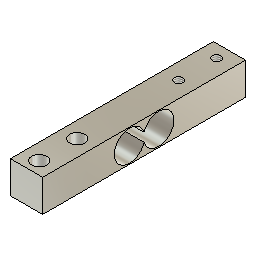
vibroDoser (Autodesk Fusion 360 archive; units mm, degrees)
design "LoadCell"
Autodesk Fusion 360 part; units mm, degrees
(part 1 of 2)
sketch "Skizze2" plane through (0, 0, 0) normal (0, 1, 0) x (1, 0, 0)
  line L0 (-6.35, -6.35) -> (6.35, -6.35)
  line L1 (6.35, -6.35) -> (6.35, 6.35)
  line L2 (6.35, 6.35) -> (-6.35, 6.35)
  line L3 (-6.35, 6.35) -> (-6.35, -6.35)
  line L4 (-6.35, -6.35) -> (6.35, 6.35) construction
  line L5 (6.35, -6.35) -> (-6.35, 6.35) construction
  dimension "d1" = 12.7
  dimension "d2" = 12.7
  constraint horizontal L0
  constraint perpendicular L0 L1
  constraint parallel L0 L2
  constraint parallel L1 L3
  constraint coincident L4 origin
  constraint coincident L5 origin
  measures "d1" distance of L1.end L2.end
  measures "d2" distance of L0.end L1.end
extrude "Extrusion1" add sketch "Skizze2" along normal blind 80
sketch "Skizze3" plane through (6.35, 0, 0) normal (1, 0, 0) x (0, 1, 0)
  line L0 (0, 6.35) -> (0, -6.35)
  line L1 (0, -6.35) -> (80, -6.35)
  line L2 (80, -6.35) -> (80, 6.35)
  line L3 (80, 6.35) -> (0, 6.35)
  line L4 (0, 0) -> (85.7645, 0) construction
  circle A0 centre (34.25, 0) radius 6
  circle A1 centre (45.75, 0) radius 6
  line L5 (40, -6.35) -> (40, 14.7485) construction
  dimension "d5" = 11.5
  dimension "d6" = 12
  dimension "d7" = 12
  dimension "d8" = 5.75
  constraint coincident L4.start origin
  constraint perpendicular L0 L4
  constraint coincident L4 A0.centre
  constraint coincident L4 A1.centre
  constraint midpoint L1 L5.start
  constraint perpendicular L3 L5
  measures "d5" distance of A0.centre A1.centre
  measures "d6" diameter of A1
  measures "d7" diameter of A0
  measures "d8" distance of A0.centre L5
extrude "Extrusion2" cut sketch "Skizze3" against normal blind 27 contours A0 A1 | A0 A1 | A0 A1
sketch "Skizze4" plane through (0, 0, 6.35) normal (0, 0, 1) x (-1, 0, 0)
  line L0 (6.35, 0) -> (-6.35, 0)
  line L1 (-6.35, 0) -> (-6.35, -80)
  line L2 (-6.35, -80) -> (6.35, -80)
  line L3 (6.35, -80) -> (6.35, 0)
  line L4 (0, 5.2844) -> (0, -87.2424)
  point P0 (0, -5)
  point P1 (0, -20)
  point P2 (0, -60)
  point P3 (0, -75)
  dimension "d11" = 5
  dimension "d12" = 15
  dimension "d13" = 15
  dimension "d14" = 5
  constraint perpendicular L2 L4
  constraint coincident origin L4
  constraint coincident L4 P0
  constraint coincident L4 P1
  constraint coincident L4 P2
  constraint coincident L4 P3
  measures "d11" distance of L0 P0
  measures "d12" distance of P0 P1
  measures "d13" distance of P2 P3
  measures "d14" distance of L2 P3
hole "Bohrung1" at (0, 5, 6.35) at (0, 20, 6.35) direction (0, 0, -1) diameter 6 depth 30 tip angle 118
hole "Bohrung2" at (0, 60, 6.35) at (0, 75, 6.35) direction (0, 0, -1) diameter 3.332 depth 30 tip angle 118
thread "Gewinde2" "ISO Metric profile 4.0 M4x0.7 6H"
equation "d8 = ( 11.5 / 2 ) * 1 mm"

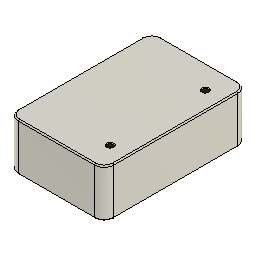
design "Schaltschrank"
Autodesk Fusion 360 part; units mm, degrees
sketch "Skizze1" plane through (0, 0, 0) normal (0, 0, 1) x (1, 0, 0)
  line L0 (-200, 300) -> (200, 300)
  line L1 (200, 300) -> (200, -300)
  line L2 (200, -300) -> (-200, -300)
  line L3 (-200, -300) -> (-200, 300)
  line L4 (-200, 300) -> (200, -300) construction
  line L5 (200, 300) -> (-200, -300) construction
  dimension "d1" = 600
  dimension "d2" = 400
  constraint horizontal L0
  constraint perpendicular L0 L1
  constraint parallel L0 L2
  constraint parallel L1 L3
  constraint coincident L4 origin
  constraint coincident L5 origin
  measures "d1" distance of L0.end L1.end
  measures "d2" distance of L0.start L0.end
extrude "Extrusion1" add sketch "Skizze1" along normal blind 200
fillet "Abrundung1" radius 40 4 edges at (200, -300, 100) (-200, -300, 100) (200, 300, 100) (-200, 300, 100)
fillet "Abrundung2" radius 5 2 faces at (-66.6667, -86.6667, 200) (-66.6667, -86.6667, 0)
sketch "Skizze2" plane through (0, 0, 200) normal (0, 0, 1) x (-1, 0, 0)
  arc A0 (160, -295) -> (195, -260) centre (160, -260) ccw
  line L0 (195, -260) -> (195, 260)
  arc A1 (195, 260) -> (160, 295) centre (160, 260) ccw
  line L1 (160, 295) -> (-160, 295)
  arc A2 (-160, 295) -> (-195, 260) centre (-160, 260) ccw
  line L2 (-195, 260) -> (-195, -260)
  arc A3 (-195, -260) -> (-160, -295) centre (-160, -260) ccw
  line L3 (-160, -295) -> (160, -295)
  line L4 (-125, -200) -> (125, -200)
  line L5 (125, -200) -> (125, 200)
  line L6 (125, 200) -> (-125, 200)
  line L7 (-125, 200) -> (-125, -200)
  line L8 (-125, -200) -> (125, 200) construction
  line L9 (125, -200) -> (-125, 200) construction
  dimension "d9" = 250
  dimension "d10" = 400
  constraint horizontal L4
  constraint perpendicular L4 L5
  constraint parallel L4 L6
  constraint parallel L5 L7
  constraint coincident L8 origin
  constraint coincident L9 origin
  measures "d9" distance of L4.start L4.end
  measures "d10" distance of L4.start L6.end
hole "Bohrung1" at (125, 200, 200) at (125, -200, 200) direction (0, 0, -1) diameter 30 depth 5 tip angle 180

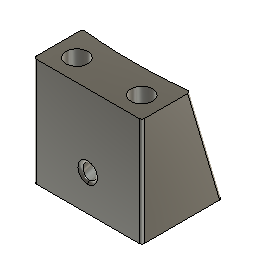
design "FunnelHolder"
Autodesk Fusion 360 part; units mm, degrees
sketch "Skizze1" plane through (0, 0, 0) normal (0, 0, 1) x (1, 0, 0)
  line L0 (-20, 20) -> (20, 20)
  line L1 (20, 20) -> (20, -20)
  line L2 (20, -20) -> (-20, -20)
  line L3 (-20, -20) -> (-20, 20)
  line L4 (-20, 20) -> (20, -20) construction
  line L5 (20, 20) -> (-20, -20) construction
  dimension "d1" = 40
  dimension "d2" = 40
  constraint horizontal L0
  constraint perpendicular L0 L1
  constraint parallel L0 L2
  constraint parallel L1 L3
  constraint coincident L4 origin
  constraint coincident L5 origin
  measures "d1" distance of L1.end L2.end
  measures "d2" distance of L0.end L1.end
extrude "Extrusion1" add sketch "Skizze1" along normal blind 40
sketch "Skizze2" plane through (0, 0, 40) normal (0, 0, 1) x (-1, 0, 0)
  line L0 (20, 20) -> (-20, 20)
  line L1 (-20, 20) -> (-20, -20)
  line L2 (-20, -20) -> (20, -20)
  line L3 (20, -20) -> (20, 20)
  circle A0 centre (0, -176) radius 179
  line L4 (0, 0) -> (0, -239.3614) construction
  dimension "d8" = 358
  dimension "d26" = 156
  constraint coincident L4.start origin
  constraint perpendicular L2 L4
  constraint coincident A0.centre L4
  measures "d8" diameter of A0
  measures "d26" distance of L2 A0.centre
ref_plane "Arbeitsebene1" through (0, 0, -340) normal (0, 0, 1) x (1, 0, 0)
sketch "Skizze3" plane through (0, 0, -340) normal (0, 0, 1) x (1, 0, 0)
  circle A0 centre (0, 176) radius 179
  circle A1 centre (0, 176) radius 67.5
  dimension "d9" = 135
  constraint concentric A0 A1
  measures "d9" diameter of A1
loft "Erhebung1" cut profiles "Skizze3", "Skizze2" section 1 contours A1 section 2 contours L1 L2 L3 A0 | L1 L2 L3 A0
ref_plane "Arbeitsebene2" through (20, -1.8792, 40) normal (0, -0.959032, -0.283299) x (1, 0, 0)
sketch "Skizze4" plane through (20, -1.8792, 40) normal (0, -0.959032, -0.283299) x (1, 0, 0)
  line L0 (0, -41.7087) -> (0, 0)
  ellipse E0 centre (-20, -88.7542) end of major axis (147.2632, -88.7542) minor radius 47.3855 (0, -41.7087) -> (-40, -41.7087) ccw
  line L1 (-40, 0) -> (-40, -41.7087)
  ellipse E1 centre (-20, -50.393) end of major axis (-199, -50.393) minor radius 50.7105 (0, 0) -> (-40, 0) ccw
  line L2 (-40, -41.7087) -> (0, 0) construction
  line L3 (0, -41.7087) -> (-40, 0) construction
  line L4 (-20, -20.8544) -> (-20, 7.4444) construction
  circle A0 centre (-20, -20.8544) radius 2.6
  point P0 (-20, -20.8544)
  dimension "d11" = 5.2
  constraint coincident L1.end L2.start
  constraint coincident L0.end L2.end
  constraint coincident L0.start L3.start
  constraint coincident L1.start L3.end
  constraint midpoint L3 P0
  constraint vertical L4
  constraint coincident L4 P0
  constraint coincident P0 L4.start
  measures "d11" diameter of A0
extrude "Extrusion2" cut sketch "Skizze4" along normal blind 40 contours A0
sketch "Skizze5" plane through (0, 0, 0) normal (0, 0, -1) x (1, 0, 0)
  arc A0 (20, -9.9369) -> (-20, -9.9369) centre (0, -176) ccw
  line L0 (20, -9.9369) -> (20, 20)
  line L1 (20, 20) -> (-20, 20)
  line L2 (-20, 20) -> (-20, -9.9369)
  line L3 (-12, 12) -> (12, 12)
  dimension "d14" = 12
  dimension "d15" = 24
  dimension "d16" = 12
  constraint perpendicular L2 L3
  measures "d14" distance of origin L3
  measures "d15" distance of L3.start L3.end
  measures "d16" horizontal distance of origin L3.start
hole "Bohrung1" at (12, -12, 0) at (-12, -12, 0) direction (0, 0, 1) diameter 8 depth 47 tip angle 118 counterbore diameter 12 counterbore depth 31
fillet "Abrundung1" radius 1 6 edges at (20, 4.129, 19.6564) (-20, 4.129, 19.6564) (20, -20, 20) (-20, -20, 20) (2.6, 2.9758, 19.7005) (0, -20, 10.1908)
fillet "Abrundung2" radius 3 2 edges at (17.594, -9.8303, 31) (-6.406, -9.8303, 31)
named bodies: "FunnelHolder"

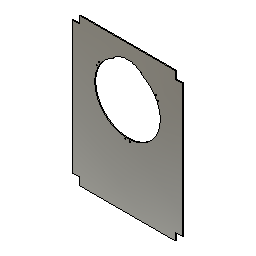
design "FrameFunnelPlate"
Autodesk Fusion 360 part; units mm, degrees
sketch "Skizze1" plane through (0, 0, 0) normal (0, 1, 0) x (1, 0, 0)
  line L0 (-300, 400) -> (300, 400)
  line L1 (300, 400) -> (300, -400)
  line L2 (300, -400) -> (-300, -400)
  line L3 (-300, -400) -> (-300, 400)
  line L4 (-300, 400) -> (300, -400) construction
  line L5 (300, 400) -> (-300, -400) construction
  line L6 (0, 273.6534) -> (0, -137.7109) construction
  circle A0 centre (0, -130) radius 177.5
  line L7 (-300, -400) -> (-259.5, -400)
  line L8 (-259.5, -400) -> (-259.5, -359.5)
  line L9 (-259.5, -359.5) -> (-300, -359.5)
  line L10 (-300, -359.5) -> (-300, -400)
  line L11 (-300, 400) -> (-259.5, 400)
  line L12 (-259.5, 400) -> (-259.5, 359.5)
  line L13 (-259.5, 359.5) -> (-300, 359.5)
  line L14 (-300, 359.5) -> (-300, 400)
  line L15 (300, 400) -> (259.5, 400)
  line L16 (259.5, 400) -> (259.5, 359.5)
  line L17 (259.5, 359.5) -> (300, 359.5)
  line L18 (300, 359.5) -> (300, 400)
  line L19 (300, -400) -> (259.5, -400)
  line L20 (259.5, -400) -> (259.5, -359.5)
  line L21 (259.5, -359.5) -> (300, -359.5)
  line L22 (300, -359.5) -> (300, -400)
  dimension "d1" = 600
  dimension "d2" = 800
  dimension "d7" = 355
  dimension "d22" = 270
  dimension "d38" = 40.5
  dimension "d39" = 40.5
  constraint horizontal L0
  constraint perpendicular L0 L1
  constraint parallel L0 L2
  constraint parallel L1 L3
  constraint coincident L4 origin
  constraint coincident L5 origin
  constraint vertical L6
  constraint coincident origin L6
  constraint coincident L6 A0.centre
  constraint horizontal L7
  constraint vertical L8
  constraint horizontal L9
  constraint vertical L10
  constraint horizontal L11
  constraint vertical L12
  constraint horizontal L13
  constraint vertical L14
  constraint horizontal L15
  constraint vertical L16
  constraint horizontal L17
  constraint vertical L18
  constraint horizontal L19
  constraint vertical L20
  constraint horizontal L21
  constraint vertical L22
  constraint equal L17 L21
  constraint equal L16 L17
  constraint equal L12 L16
  constraint equal L12 L13
  constraint equal L9 L12
  constraint equal L8 L9
  measures "d1" distance of L1.end L2.end
  measures "d2" distance of L0.end L1.end
  measures "d7" diameter of A0
  measures "d22" distance of L2 A0.centre
  measures "d38" distance of L1.end L19.end
  measures "d39" distance of L1.end L21.end
extrude "Extrusion1" add sketch "Skizze1" along normal blind 5 contours L0 L1 L2 L3 L8 L9 L12 L13 L16 L17 L20 L21
sketch "Skizze3" plane through (0, 0, 0) normal (0, -1, 0) x (1, 0, 0)
  circle A0 centre (0, 130) radius 177.5
  line L0 (259.5, 400) -> (-259.5, 400)
  line L1 (-300, 359.5) -> (-300, -359.5)
  line L2 (-259.5, -400) -> (259.5, -400)
  line L3 (300, -359.5) -> (300, 359.5)
  circle A1 centre (0, 130) radius 177.5
  line L4 (-75, 312.5) -> (75, 312.5)
  line L5 (75, 312.5) -> (75, -52.5)
  line L6 (75, -52.5) -> (-75, -52.5)
  line L7 (-75, -52.5) -> (-75, 312.5)
  line L8 (-75, 312.5) -> (75, -52.5) construction
  line L9 (75, 312.5) -> (-75, -52.5) construction
  circle A2 centre (0, 130) radius 182.5
  line L10 (-25, 322.5) -> (25, 322.5)
  line L11 (25, 322.5) -> (25, -62.5)
  line L12 (25, -62.5) -> (-25, -62.5)
  line L13 (-25, -62.5) -> (-25, 322.5)
  line L14 (-25, 322.5) -> (25, -62.5) construction
  line L15 (25, 322.5) -> (-25, -62.5) construction
  circle A3 centre (0, 201.7754) radius 120.7246
  line L16 (259.5, 359.5) -> (259.5, 400)
  line L17 (-259.5, 400) -> (-259.5, 359.5)
  line L18 (-259.5, 359.5) -> (-300, 359.5)
  line L19 (-300, -359.5) -> (-259.5, -359.5)
  line L20 (-259.5, -359.5) -> (-259.5, -400)
  line L21 (259.5, -400) -> (259.5, -359.5)
  line L22 (259.5, -359.5) -> (300, -359.5)
  line L23 (300, 359.5) -> (259.5, 359.5)
  point P0 (0, 130)
  point P1 (0, 130)
  point P2 (-75, 296.3768)
  point P3 (75, 296.3768)
  dimension "d30" = 150
  dimension "d31" = 365
  dimension "d32" = 50
  dimension "d33" = 10
  constraint horizontal L4
  constraint perpendicular L4 L5
  constraint parallel L4 L6
  constraint parallel L5 L7
  constraint coincident L8 P1
  constraint coincident L9 P1
  constraint coincident P1 P0
  constraint tangent L4 A2
  constraint horizontal L10
  constraint perpendicular L10 L11
  constraint parallel L10 L12
  constraint parallel L11 L13
  constraint coincident L14 P1
  constraint coincident L15 P1
  constraint tangent L10 A3
  constraint coincident L7 P2
  constraint coincident A2 P2
  constraint coincident L5 P3
  constraint coincident A2 P3
  constraint coincident A3 P2
  constraint coincident A3 P3
  measures "d30" distance of L4.start L4.end
  measures "d31" diameter of A2
  measures "d32" distance of L10.start L10.end
  measures "d33" distance of L4 L10
extrude "Extrusion2" cut sketch "Skizze3" against normal blind 20 contours A0 A1 L5 A2 L11 | L4 A2 L11 A3 | A0 A1 A2 L11 L13 | L4 A2 L11 | L4 L11 A3 | A0 A1 L7 A2 L13 | L4 A2 L13 | L4 L11 L13 A3 | L10 L11 A3 | L4 A2 L13 A3 | L4 L13 A3 | L10 L13 A3 picked at (69.6159, 294.9048) picked at (0, 309.0354) picked at (-69.6159, 294.9048)
fillet "Abrundung2" radius 2 8 edges at (-75, 2.5, 290.8765) (-25, 2.5, 322.5) (25, 2.5, 322.5) (75, 2.5, 290.8765) (-25, 2.5, 319.8831) (25, 2.5, 319.8831) (75, 2.5, 296.3768) (-75, 2.5, 296.3768)
fillet "Abrundung3" radius 2 12 edges at (-300, 2.5, -359.5) (-259.5, 2.5, -359.5) (-259.5, 2.5, -400) (259.5, 2.5, -400) (259.5, 2.5, -359.5) (300, 2.5, -359.5) (-300, 2.5, 359.5) (-259.5, 2.5, 359.5) (-259.5, 2.5, 400) (259.5, 2.5, 400) (259.5, 2.5, 359.5) (300, 2.5, 359.5)
sketch "Skizze5" plane through (0, 0, 0) normal (0, -1, 0) x (1, 0, 0)
  arc A0 (25.0626, 320.9965) -> (26.56, 319.5421) centre (27, 321.4931) ccw
  arc A1 (74.2297, 296.9824) -> (26.56, 319.5421) centre (0, 201.7754) ccw
  arc A2 (75, 295.4052) -> (74.2297, 296.9824) centre (73, 295.4052) ccw
  line L0 (75, 295.4052) -> (75, 292.1458)
  arc A3 (75, 292.1458) -> (76.1421, 290.3391) centre (77, 292.1458) ccw
  arc A4 (-76.1421, 290.3391) -> (76.1421, 290.3391) centre (0, 130) ccw
  arc A5 (-76.1421, 290.3391) -> (-75, 292.1458) centre (-77, 292.1458) ccw
  line L1 (-75, 292.1458) -> (-75, 295.4052)
  arc A6 (-74.2297, 296.9824) -> (-75, 295.4052) centre (-73, 295.4052) ccw
  arc A7 (-26.56, 319.5421) -> (-74.2297, 296.9824) centre (0, 201.7754) ccw
  arc A8 (-26.56, 319.5421) -> (-25.0626, 320.9965) centre (-27, 321.4931) ccw
  arc A9 (-23.1252, 322.5) -> (-25.0626, 320.9965) centre (-23.1252, 320.5) ccw
  line L2 (-23.1252, 322.5) -> (23.1252, 322.5)
  arc A10 (25.0626, 320.9965) -> (23.1252, 322.5) centre (23.1252, 320.5) ccw
  arc A11 (300, 357.5) -> (298, 359.5) centre (298, 357.5) ccw
  line L3 (298, 359.5) -> (261.5, 359.5)
  arc A12 (259.5, 361.5) -> (261.5, 359.5) centre (261.5, 361.5) ccw
  line L4 (259.5, 361.5) -> (259.5, 398)
  arc A13 (259.5, 398) -> (257.5, 400) centre (257.5, 398) ccw
  line L5 (257.5, 400) -> (-257.5, 400)
  arc A14 (-257.5, 400) -> (-259.5, 398) centre (-257.5, 398) ccw
  line L6 (-259.5, 398) -> (-259.5, 361.5)
  arc A15 (-261.5, 359.5) -> (-259.5, 361.5) centre (-261.5, 361.5) ccw
  line L7 (-261.5, 359.5) -> (-298, 359.5)
  arc A16 (-298, 359.5) -> (-300, 357.5) centre (-298, 357.5) ccw
  line L8 (-300, 357.5) -> (-300, -357.5)
  arc A17 (-300, -357.5) -> (-298, -359.5) centre (-298, -357.5) ccw
  line L9 (-298, -359.5) -> (-261.5, -359.5)
  arc A18 (-259.5, -361.5) -> (-261.5, -359.5) centre (-261.5, -361.5) ccw
  line L10 (-259.5, -361.5) -> (-259.5, -398)
  arc A19 (-259.5, -398) -> (-257.5, -400) centre (-257.5, -398) ccw
  line L11 (-257.5, -400) -> (257.5, -400)
  arc A20 (257.5, -400) -> (259.5, -398) centre (257.5, -398) ccw
  line L12 (259.5, -398) -> (259.5, -361.5)
  arc A21 (261.5, -359.5) -> (259.5, -361.5) centre (261.5, -361.5) ccw
  line L13 (261.5, -359.5) -> (298, -359.5)
  arc A22 (298, -359.5) -> (300, -357.5) centre (298, -357.5) ccw
  line L14 (300, -357.5) -> (300, 357.5)
  arc A23 (-76.1421, 290.3391) -> (76.1421, 290.3391) centre (0, 130) ccw
  circle A24 centre (0, 130) radius 186.5
  line L15 (0, -56.5) -> (0, 440.8023)
  line L16 (-161.5137, 223.25) -> (161.5137, 36.75)
  line L17 (-161.5137, 36.75) -> (161.5137, 223.25)
  line L18 (-167.5137, 212.8577) -> (-155.5137, 233.6423)
  line L19 (155.5137, 233.6423) -> (167.5137, 212.8577)
  line L20 (-12, -56.5) -> (12, -56.5)
  point P0 (-161.5137, 223.25)
  point P1 (161.5137, 223.25)
  point P2 (0, -56.5)
  dimension "d42" = 373
  dimension "d43" = 120
  dimension "d44" = 120
  dimension "d49" = 24
  dimension "d52" = 24
  dimension "d53" = 12
  dimension "d54" = 24
  dimension "d55" = 12
  dimension "d56" = 12
  constraint concentric A23 A24
  constraint coincident A24 P2
  constraint perpendicular L5 L15
  constraint coincident A24 P0
  constraint coincident A24 L16.end
  constraint coincident A4.centre L16
  constraint coincident A24 L17.start
  constraint coincident A24 P1
  constraint coincident A4.centre L17
  constraint coincident A4.centre L15
  constraint coincident P0 L16.start
  constraint coincident P1 L17.end
  constraint coincident P2 L15.start
  constraint tangent A24 L18
  constraint coincident P0 L18
  constraint tangent A24 L19
  constraint coincident P1 L19
  constraint tangent A24 L20
  constraint coincident P2 L20
  measures "d42" diameter of A24
  measures "d43" angle of L15 L16
  measures "d44" angle of L15 L17
  measures "d49" distance of L18.start L18.end
  measures "d52" distance of L19.start L19.end
  measures "d53" distance of P1 L19.start
  measures "d54" distance of L20.start L20.end
  measures "d55" distance of P2 L20.start
  measures "d56" distance of P0 L18.start
hole "Bohrung2" at (-12, 0, -56.5) at (12, 0, -56.5) at (-167.5137, 0, 212.8577) at (-155.5137, 0, 233.6423) at (167.5137, 0, 212.8577) at (155.5137, 0, 233.6423) direction (0, 1, 0) diameter 6.8 depth 5 tip angle 118
sketch "Skizze6" plane through (0, 0, 0) normal (0, -1, 0) x (1, 0, 0)
  arc A0 (25.0626, 320.9965) -> (26.56, 319.5421) centre (27, 321.4931) ccw
  arc A1 (74.2297, 296.9824) -> (26.56, 319.5421) centre (0, 201.7754) ccw
  arc A2 (75, 295.4052) -> (74.2297, 296.9824) centre (73, 295.4052) ccw
  line L0 (75, 295.4052) -> (75, 292.1458)
  arc A3 (75, 292.1458) -> (76.1421, 290.3391) centre (77, 292.1458) ccw
  arc A4 (-76.1421, 290.3391) -> (76.1421, 290.3391) centre (0, 130) ccw
  arc A5 (-76.1421, 290.3391) -> (-75, 292.1458) centre (-77, 292.1458) ccw
  line L1 (-75, 292.1458) -> (-75, 295.4052)
  arc A6 (-74.2297, 296.9824) -> (-75, 295.4052) centre (-73, 295.4052) ccw
  arc A7 (-26.56, 319.5421) -> (-74.2297, 296.9824) centre (0, 201.7754) ccw
  arc A8 (-26.56, 319.5421) -> (-25.0626, 320.9965) centre (-27, 321.4931) ccw
  arc A9 (-23.1252, 322.5) -> (-25.0626, 320.9965) centre (-23.1252, 320.5) ccw
  line L2 (-23.1252, 322.5) -> (23.1252, 322.5)
  arc A10 (25.0626, 320.9965) -> (23.1252, 322.5) centre (23.1252, 320.5) ccw
  arc A11 (300, 357.5) -> (298, 359.5) centre (298, 357.5) ccw
  line L3 (298, 359.5) -> (261.5, 359.5)
  arc A12 (259.5, 361.5) -> (261.5, 359.5) centre (261.5, 361.5) ccw
  line L4 (259.5, 361.5) -> (259.5, 398)
  arc A13 (259.5, 398) -> (257.5, 400) centre (257.5, 398) ccw
  line L5 (257.5, 400) -> (-257.5, 400)
  arc A14 (-257.5, 400) -> (-259.5, 398) centre (-257.5, 398) ccw
  line L6 (-259.5, 398) -> (-259.5, 361.5)
  arc A15 (-261.5, 359.5) -> (-259.5, 361.5) centre (-261.5, 361.5) ccw
  line L7 (-261.5, 359.5) -> (-298, 359.5)
  arc A16 (-298, 359.5) -> (-300, 357.5) centre (-298, 357.5) ccw
  line L8 (-300, 357.5) -> (-300, -357.5)
  arc A17 (-300, -357.5) -> (-298, -359.5) centre (-298, -357.5) ccw
  line L9 (-298, -359.5) -> (-261.5, -359.5)
  arc A18 (-259.5, -361.5) -> (-261.5, -359.5) centre (-261.5, -361.5) ccw
  line L10 (-259.5, -361.5) -> (-259.5, -398)
  arc A19 (-259.5, -398) -> (-257.5, -400) centre (-257.5, -398) ccw
  line L11 (-257.5, -400) -> (257.5, -400)
  arc A20 (257.5, -400) -> (259.5, -398) centre (257.5, -398) ccw
  line L12 (259.5, -398) -> (259.5, -361.5)
  arc A21 (261.5, -359.5) -> (259.5, -361.5) centre (261.5, -361.5) ccw
  line L13 (261.5, -359.5) -> (298, -359.5)
  arc A22 (298, -359.5) -> (300, -357.5) centre (298, -357.5) ccw
  line L14 (300, -357.5) -> (300, 357.5)
  circle A23 centre (167.5137, 212.8577) radius 3.4
  circle A24 centre (-167.5137, 212.8577) radius 3.4
  circle A25 centre (-12, -56.5) radius 3.4
  circle A26 centre (12, -56.5) radius 3.4
  circle A27 centre (-155.5137, 233.6423) radius 3.4
  circle A28 centre (155.5137, 233.6423) radius 3.4
sketch "Skizze4" plane through (0, 0, 0) normal (0, -1, 0) x (1, 0, 0)
  arc A0 (75, 293.8048) -> (76.1492, 291.9948) centre (77, 293.8048) ccw
  arc A1 (-76.1492, 291.9948) -> (76.1492, 291.9948) centre (0, 130) ccw
  arc A2 (-76.1492, 291.9948) -> (-75, 293.8048) centre (-77, 293.8048) ccw
  arc A3 (-23.1252, 322.5) -> (-25.0626, 320.9965) centre (-23.1252, 320.5) ccw
  line L0 (-23.1252, 322.5) -> (23.1252, 322.5)
  arc A4 (25.0626, 320.9965) -> (23.1252, 322.5) centre (23.1252, 320.5) ccw
  line L1 (257.5, 400) -> (-257.5, 400)
  line L2 (-300, 357.5) -> (-300, -357.5)
  line L3 (-257.5, -400) -> (257.5, -400)
  line L4 (300, -357.5) -> (300, 357.5)
  line L5 (-75, 293.8048) -> (-75, 295.4052)
  line L6 (75, 295.4052) -> (75, 293.8048)
  arc A5 (-26.56, 319.5421) -> (-74.2297, 296.9824) centre (0, 201.7754) ccw
  arc A6 (74.2297, 296.9824) -> (26.56, 319.5421) centre (0, 201.7754) ccw
  arc A7 (25.0626, 320.9965) -> (26.56, 319.5421) centre (27, 321.4931) ccw
  arc A8 (75, 295.4052) -> (74.2297, 296.9824) centre (73, 295.4052) ccw
  arc A9 (-74.2297, 296.9824) -> (-75, 295.4052) centre (-73, 295.4052) ccw
  arc A10 (-26.56, 319.5421) -> (-25.0626, 320.9965) centre (-27, 321.4931) ccw
  line L7 (259.5, 361.5) -> (259.5, 398)
  line L8 (-259.5, 398) -> (-259.5, 361.5)
  line L9 (-261.5, 359.5) -> (-298, 359.5)
  line L10 (-298, -359.5) -> (-261.5, -359.5)
  line L11 (-259.5, -361.5) -> (-259.5, -398)
  line L12 (259.5, -398) -> (259.5, -361.5)
  line L13 (261.5, -359.5) -> (298, -359.5)
  line L14 (298, 359.5) -> (261.5, 359.5)
  arc A11 (300, 357.5) -> (298, 359.5) centre (298, 357.5) ccw
  arc A12 (259.5, 361.5) -> (261.5, 359.5) centre (261.5, 361.5) ccw
  arc A13 (259.5, 398) -> (257.5, 400) centre (257.5, 398) ccw
  arc A14 (-257.5, 400) -> (-259.5, 398) centre (-257.5, 398) ccw
  arc A15 (-261.5, 359.5) -> (-259.5, 361.5) centre (-261.5, 361.5) ccw
  arc A16 (-298, 359.5) -> (-300, 357.5) centre (-298, 357.5) ccw
  arc A17 (-300, -357.5) -> (-298, -359.5) centre (-298, -357.5) ccw
  arc A18 (-259.5, -361.5) -> (-261.5, -359.5) centre (-261.5, -361.5) ccw
  arc A19 (-259.5, -398) -> (-257.5, -400) centre (-257.5, -398) ccw
  arc A20 (257.5, -400) -> (259.5, -398) centre (257.5, -398) ccw
  arc A21 (261.5, -359.5) -> (259.5, -361.5) centre (261.5, -361.5) ccw
  arc A22 (298, -359.5) -> (300, -357.5) centre (298, -357.5) ccw

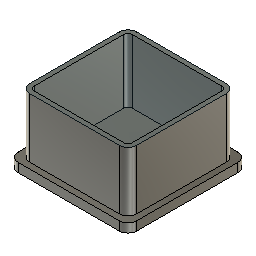
design "PipeCover4040"
Autodesk Fusion 360 part; units mm, degrees
sketch "Skizze1" plane through (0, 0, 0) normal (0, 0, 1) x (1, 0, 0)
  line L0 (-20, 20) -> (20, 20)
  line L1 (20, 20) -> (20, -20)
  line L2 (20, -20) -> (-20, -20)
  line L3 (-20, -20) -> (-20, 20)
  line L4 (-20, 20) -> (20, -20) construction
  line L5 (20, 20) -> (-20, -20) construction
  dimension "d1" = 40
  dimension "d2" = 40
  constraint horizontal L0
  constraint perpendicular L0 L1
  constraint parallel L0 L2
  constraint parallel L1 L3
  constraint coincident L4 origin
  constraint coincident L5 origin
  measures "d1" distance of L1.end L2.end
  measures "d2" distance of L0.end L1.end
extrude "Extrusion1" add sketch "Skizze1" along normal blind 3
sketch "Skizze2" plane through (0, 0, 3) normal (0, 0, 1) x (-1, 0, 0)
  line L0 (20, 20) -> (-20, 20)
  line L1 (-20, 20) -> (-20, -20)
  line L2 (-20, -20) -> (20, -20)
  line L3 (20, -20) -> (20, 20)
  line L4 (18, -18) -> (-18, -18)
  line L5 (-18, -18) -> (-18, 18)
  line L6 (-18, 18) -> (18, 18)
  line L7 (18, 18) -> (18, -18)
  line L8 (18, -18) -> (-18, 18) construction
  line L9 (-18, -18) -> (18, 18) construction
  dimension "d5" = 2
  dimension "d6" = 2
  constraint horizontal L4
  constraint perpendicular L4 L5
  constraint parallel L4 L6
  constraint parallel L5 L7
  constraint coincident L8 origin
  constraint coincident L9 origin
  measures "d5" distance of L3 L7
  measures "d6" distance of L2 L4
extrude "Extrusion2" add sketch "Skizze2" along normal blind 20 contours L4 L5 L6 L7
fillet "Abrundung1" radius 3 8 edges at (-20, -20, 1.5) (-18, -18, 13) (20, -20, 1.5) (18, -18, 13) (18, 18, 13) (20, 20, 1.5) (-18, 18, 13) (-20, 20, 1.5)
sketch "Skizze3" plane through (0, 0, 23) normal (0, 0, 1) x (-1, 0, 0)
  arc A0 (15, -18) -> (18, -15) centre (15, -15) ccw
  line L0 (18, -15) -> (18, 15)
  arc A1 (18, 15) -> (15, 18) centre (15, 15) ccw
  line L1 (15, 18) -> (-15, 18)
  arc A2 (-15, 18) -> (-18, 15) centre (-15, 15) ccw
  line L2 (-18, 15) -> (-18, -15)
  arc A3 (-18, -15) -> (-15, -18) centre (-15, -15) ccw
  line L3 (-15, -18) -> (15, -18)
shell "Schale1" thickness 1.5 removed faces 1 at (4, -5, 23)
named bodies: "PipeCover"

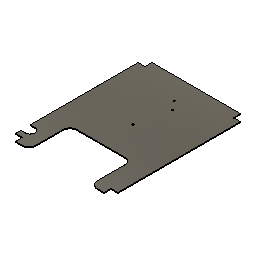
design "FrameMidPlate"
Autodesk Fusion 360 part; units mm, degrees
sketch "Skizze1" plane through (0, 0, 0) normal (0, 0, 1) x (1, 0, 0)
  line L0 (-300, 400) -> (300, 400)
  line L1 (300, 400) -> (300, -400)
  line L2 (300, -400) -> (-300, -400)
  line L3 (-300, -400) -> (-300, 400)
  line L4 (-300, 400) -> (300, -400) construction
  line L5 (300, 400) -> (-300, -400) construction
  line L6 (-259.5, 359.5) -> (259.5, 359.5)
  line L7 (259.5, 359.5) -> (259.5, -359.5)
  line L8 (259.5, -359.5) -> (-259.5, -359.5)
  line L9 (-259.5, -359.5) -> (-259.5, 359.5)
  line L10 (-259.5, 359.5) -> (259.5, -359.5) construction
  line L11 (259.5, 359.5) -> (-259.5, -359.5) construction
  line L12 (-300, 400) -> (-259.5, 400)
  line L13 (-259.5, 400) -> (-259.5, 359.5)
  line L14 (-259.5, 359.5) -> (-300, 359.5)
  line L15 (-300, 359.5) -> (-300, 400)
  line L16 (259.5, 359.5) -> (300, 359.5)
  line L17 (300, 359.5) -> (300, 400)
  line L18 (300, 400) -> (259.5, 400)
  line L19 (259.5, 400) -> (259.5, 359.5)
  line L20 (-259.5, -359.5) -> (-300, -359.5)
  line L21 (-300, -359.5) -> (-300, -400)
  line L22 (-300, -400) -> (-259.5, -400)
  line L23 (-259.5, -400) -> (-259.5, -359.5)
  line L24 (259.5, -359.5) -> (300, -359.5)
  line L25 (300, -359.5) -> (300, -400)
  line L26 (300, -400) -> (259.5, -400)
  line L27 (259.5, -400) -> (259.5, -359.5)
  dimension "d1" = 600
  dimension "d2" = 800
  dimension "d3" = 40.5
  dimension "d4" = 40.5
  constraint horizontal L0
  constraint perpendicular L0 L1
  constraint parallel L0 L2
  constraint parallel L1 L3
  constraint coincident L4 origin
  constraint coincident L5 origin
  constraint horizontal L6
  constraint perpendicular L6 L7
  constraint parallel L6 L8
  constraint parallel L7 L9
  constraint coincident L10 origin
  constraint coincident L11 origin
  constraint horizontal L12
  constraint vertical L13
  constraint horizontal L14
  constraint vertical L15
  constraint horizontal L16
  constraint vertical L17
  constraint horizontal L18
  constraint vertical L19
  constraint horizontal L20
  constraint vertical L21
  constraint horizontal L22
  constraint vertical L23
  constraint horizontal L24
  constraint vertical L25
  constraint horizontal L26
  constraint vertical L27
  constraint coincident L0.end L17
  constraint coincident L0 L1.start
  measures "d1" distance of L1.end L2.end
  measures "d2" distance of L0.end L1.end
  measures "d3" distance of L0 L6
  measures "d4" distance of L3 L9
extrude "Extrusion1" add sketch "Skizze1" along normal blind 5 contours L0 L6 L13 L19 | L3 L9 L14 L20 | L6 L7 L8 L9 | L1 L7 L16 L24 | L2 L8 L23 L27
sketch "Skizze4" plane through (0, 0, 5) normal (0, 0, 1) x (-1, 0, 0)
  line L0 (259.5, 400) -> (-259.5, 400)
  line L1 (-259.5, 400) -> (-259.5, 359.5)
  line L2 (-259.5, 359.5) -> (-300, 359.5)
  line L3 (-300, 359.5) -> (-300, -359.5)
  line L4 (-300, -359.5) -> (-259.5, -359.5)
  line L5 (-259.5, -359.5) -> (-259.5, -400)
  line L6 (-259.5, -400) -> (259.5, -400)
  line L7 (259.5, -400) -> (259.5, -359.5)
  line L8 (259.5, -359.5) -> (300, -359.5)
  line L9 (300, -359.5) -> (300, 359.5)
  line L10 (300, 359.5) -> (259.5, 359.5)
  line L11 (259.5, 359.5) -> (259.5, 400)
  line L12 (0, -270) -> (0, -30)
  dimension "d23" = 240
  dimension "d24" = 130
  constraint vertical L12
  constraint coincident origin L12
  measures "d23" distance of L12.start L12.end
  measures "d24" distance of L6 L12.start
hole "Bohrung3" at (0, 270, 5) at (0, 30, 5) direction (0, 0, -1) diameter 10 depth 10 tip angle 118
sketch "Skizze6" plane through (0, 0, 5) normal (0, 0, 1) x (-1, 0, 0)
  line L0 (259.5, -400) -> (259.5, -359.5)
  line L1 (259.5, -359.5) -> (300, -359.5)
  line L2 (300, -359.5) -> (300, 359.5)
  line L3 (300, 359.5) -> (259.5, 359.5)
  line L4 (259.5, 359.5) -> (259.5, 400)
  line L5 (259.5, 400) -> (-259.5, 400)
  line L6 (-259.5, 400) -> (-259.5, 359.5)
  line L7 (-259.5, 359.5) -> (-300, 359.5)
  line L8 (-300, 359.5) -> (-300, -359.5)
  line L9 (-300, -359.5) -> (-259.5, -359.5)
  line L10 (-259.5, -359.5) -> (-259.5, -400)
  line L11 (-259.5, -400) -> (259.5, -400)
  circle A0 centre (0, -270) radius 5
  circle A1 centre (0, -30) radius 5
  line L12 (180, 400) -> (-180, 400)
  line L13 (-180, 400) -> (-180, 160)
  line L14 (-180, 160) -> (180, 160)
  line L15 (180, 160) -> (180, 400)
  line L16 (259.75, 160.25) -> (300.25, 160.25)
  line L17 (300.25, 160.25) -> (300.25, 119.75)
  line L18 (300.25, 119.75) -> (259.75, 119.75)
  line L19 (259.75, 119.75) -> (259.75, 160.25)
  line L20 (259.75, 160.25) -> (300.25, 119.75) construction
  line L21 (300.25, 160.25) -> (259.75, 119.75) construction
  line L22 (-300.25, 160.25) -> (-259.75, 160.25)
  line L23 (-259.75, 160.25) -> (-259.75, 119.75)
  line L24 (-259.75, 119.75) -> (-300.25, 119.75)
  line L25 (-300.25, 119.75) -> (-300.25, 160.25)
  line L26 (-300.25, 160.25) -> (-259.75, 119.75) construction
  line L27 (-259.75, 160.25) -> (-300.25, 119.75) construction
  point P0 (280, 140)
  point P1 (-280, 140)
  dimension "d30" = 560
  dimension "d31" = 120
  dimension "d32" = 120
  dimension "d37" = 40.5
  dimension "d38" = 40.5
  dimension "d39" = 20
  dimension "d40" = 20
  dimension "d42" = 20
  dimension "d43" = 20
  constraint horizontal L12
  constraint vertical L13
  constraint horizontal L14
  constraint vertical L15
  constraint coincident L5 L12.start
  constraint horizontal L16
  constraint perpendicular L16 L17
  constraint parallel L16 L18
  constraint parallel L17 L19
  constraint coincident L20 P0
  constraint coincident L21 P0
  constraint horizontal L22
  constraint perpendicular L22 L23
  constraint parallel L22 L24
  constraint parallel L23 L25
  constraint coincident L26 P1
  constraint coincident L27 P1
  constraint equal L18 L24
  constraint equal L19 L23
  measures "d30" distance of L11 L14
  measures "d31" distance of L2 L15
  measures "d32" distance of L8 L13
  measures "d37" distance of L17.end L18.end
  measures "d38" distance of L16.end L17.end
  measures "d39" distance of L2 P0
  measures "d40" distance of L8 P1
  measures "d42" distance of L14 P1
  measures "d43" distance of L14 P0
extrude "Extrusion2" cut sketch "Skizze6" against normal blind 10 contours L2 L16 L17 L18 | L8 L22 L24 L25 | L5 L12 L13 L14 L15
sketch "Skizze8" plane through (0, 0, 5) normal (0, 0, 1) x (-1, 0, 0)
  line L0 (-180, 160) -> (-180, 400)
  line L1 (-180, 400) -> (-259.5, 400)
  line L2 (-259.5, 400) -> (-259.5, 359.5)
  line L3 (-259.5, 359.5) -> (-300, 359.5)
  line L4 (-300, 359.5) -> (-300, -359.5)
  line L5 (-300, -359.5) -> (-259.5, -359.5)
  line L6 (-259.5, -359.5) -> (-259.5, -400)
  line L7 (-259.5, -400) -> (259.5, -400)
  line L8 (259.5, -400) -> (259.5, -359.5)
  line L9 (259.5, -359.5) -> (300, -359.5)
  line L10 (300, -359.5) -> (300, 359.5)
  line L11 (300, 359.5) -> (259.5, 359.5)
  line L12 (259.5, 359.5) -> (259.5, 400)
  line L13 (259.5, 400) -> (180, 400)
  line L14 (180, 400) -> (180, 160)
  line L15 (180, 160) -> (-180, 160)
  circle A0 centre (0, -270) radius 5
  circle A1 centre (0, -30) radius 5
  line L16 (0, -270) -> (-40, -270)
  line L17 (-40, -270) -> (-40, -220)
  line L18 (-40, -220) -> (0, -220)
  line L19 (0, -220) -> (0, -270)
  dimension "d44" = 40
  dimension "d45" = 50
  constraint horizontal L16
  constraint vertical L17
  constraint horizontal L18
  constraint vertical L19
  constraint coincident A0.centre L16.start
  measures "d44" distance of A0.centre L16.end
  measures "d45" distance of L16.end L17.end
hole "Bohrung4" at (40, 220, 5) direction (0, 0, -1) diameter 10 depth 50 tip angle 118
sketch "Skizze9" plane through (0, 0, 5) normal (0, 0, 1) x (-1, 0, 0)
  circle A0 centre (-40, -220) radius 5
  line L0 (-180, 160) -> (-180, 400)
  line L1 (-180, 400) -> (-259.5, 400)
  line L2 (-259.5, 400) -> (-259.5, 359.5)
  line L3 (-259.5, 359.5) -> (-300, 359.5)
  line L4 (-300, 359.5) -> (-300, -359.5)
  line L5 (-300, -359.5) -> (-259.5, -359.5)
  line L6 (-259.5, -359.5) -> (-259.5, -400)
  line L7 (-259.5, -400) -> (259.5, -400)
  line L8 (259.5, -400) -> (259.5, -359.5)
  line L9 (259.5, -359.5) -> (300, -359.5)
  line L10 (300, -359.5) -> (300, 359.5)
  line L11 (300, 359.5) -> (259.5, 359.5)
  line L12 (259.5, 359.5) -> (259.5, 400)
  line L13 (259.5, 400) -> (180, 400)
  line L14 (180, 400) -> (180, 160)
  line L15 (180, 160) -> (-180, 160)
  circle A1 centre (0, -270) radius 5
  circle A2 centre (0, -30) radius 5
  circle A3 centre (272.5, 300) radius 27.5
  line L16 (272.5, 272.5) -> (397.3448, 272.5)
  line L17 (397.3448, 272.5) -> (397.3448, 327.5)
  line L18 (397.3448, 327.5) -> (272.5, 327.5)
  line L19 (272.5, 327.5) -> (272.5, 272.5)
  dimension "d49" = 55
  dimension "d50" = 100
  dimension "d51" = 27.5
  constraint horizontal L16
  constraint vertical L17
  constraint horizontal L18
  constraint vertical L19
  constraint coincident A3 L16.start
  constraint tangent A3 L18
  constraint coincident A3.centre L19
  measures "d49" diameter of A3
  measures "d50" distance of L13 A3.centre
  measures "d51" distance of L10 A3.centre
extrude "Extrusion3" cut sketch "Skizze9" against normal blind 10 contours L10 A3 L18 | A3 L19 | L10 A3 L16 | A3 L19
fillet "Abrundung2" radius 40 4 edges at (-180, -160, 2.5) (180, -160, 2.5) (-180, -400, 2.5) (180, -400, 2.5)
fillet "Abrundung1" radius 2 12 edges at (-300, -359.5, 2.5) (-259.5, -359.5, 2.5) (-259.5, -400, 2.5) (259.5, -400, 2.5) (259.5, -359.5, 2.5) (300, -359.5, 2.5) (300, 359.5, 2.5) (259.5, 359.5, 2.5) (259.5, 400, 2.5) (-300, 359.5, 2.5) (-259.5, 359.5, 2.5) (-259.5, 400, 2.5)
sketch "Skizze7" plane through (0, 0, 5) normal (0, 0, 1) x (-1, 0, 0)
  arc A0 (257.5, -400) -> (259.5, -398) centre (257.5, -398) ccw
  line L0 (259.5, -398) -> (259.5, -361.5)
  arc A1 (261.5, -359.5) -> (259.5, -361.5) centre (261.5, -361.5) ccw
  line L1 (261.5, -359.5) -> (298, -359.5)
  arc A2 (298, -359.5) -> (300, -357.5) centre (298, -357.5) ccw
  line L2 (300, -357.5) -> (300, 272.5)
  arc A3 (300, 357.5) -> (298, 359.5) centre (298, 357.5) ccw
  line L3 (298, 359.5) -> (261.5, 359.5)
  arc A4 (259.5, 361.5) -> (261.5, 359.5) centre (261.5, 361.5) ccw
  line L4 (259.5, 361.5) -> (259.5, 398)
  arc A5 (259.5, 398) -> (257.5, 400) centre (257.5, 398) ccw
  line L5 (257.5, 400) -> (220, 400)
  arc A6 (220, 400) -> (180, 360) centre (220, 360) ccw
  line L6 (180, 360) -> (180, 200)
  arc A7 (140, 160) -> (180, 200) centre (140, 200) ccw
  line L7 (140, 160) -> (-140, 160)
  arc A8 (-180, 200) -> (-140, 160) centre (-140, 200) ccw
  line L8 (-180, 200) -> (-180, 360)
  arc A9 (-180, 360) -> (-220, 400) centre (-220, 360) ccw
  line L9 (-220, 400) -> (-257.5, 400)
  arc A10 (-257.5, 400) -> (-259.5, 398) centre (-257.5, 398) ccw
  line L10 (-259.5, 398) -> (-259.5, 361.5)
  arc A11 (-261.5, 359.5) -> (-259.5, 361.5) centre (-261.5, 361.5) ccw
  line L11 (-261.5, 359.5) -> (-298, 359.5)
  arc A12 (-298, 359.5) -> (-300, 357.5) centre (-298, 357.5) ccw
  line L12 (-300, 357.5) -> (-300, -357.5)
  arc A13 (-300, -357.5) -> (-298, -359.5) centre (-298, -357.5) ccw
  line L13 (-298, -359.5) -> (-261.5, -359.5)
  arc A14 (-259.5, -361.5) -> (-261.5, -359.5) centre (-261.5, -361.5) ccw
  line L14 (-259.5, -361.5) -> (-259.5, -398)
  arc A15 (-259.5, -398) -> (-257.5, -400) centre (-257.5, -398) ccw
  line L15 (-257.5, -400) -> (257.5, -400)
  circle A16 centre (0, -270) radius 5
  circle A17 centre (0, -30) radius 5
  circle A18 centre (-40, -220) radius 5
  line L16 (300, 272.5) -> (272.5, 272.5)
  arc A19 (272.5, 327.5) -> (272.5, 272.5) centre (272.5, 300) ccw
  line L17 (272.5, 327.5) -> (300, 327.5)
  line L18 (300, 327.5) -> (300, 357.5)

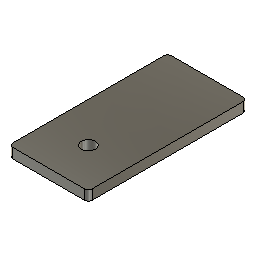
design "FootPlate"
Autodesk Fusion 360 part; units mm, degrees
sketch "Skizze1" plane through (0, 0, 0) normal (0, 0, 1) x (1, 0, 0)
  line L0 (-20, 40) -> (20, 40)
  line L1 (20, 40) -> (20, -40)
  line L2 (20, -40) -> (-20, -40)
  line L3 (-20, -40) -> (-20, 40)
  line L4 (-20, 40) -> (20, -40) construction
  line L5 (20, 40) -> (-20, -40) construction
  dimension "d1" = 40
  dimension "d2" = 80
  constraint horizontal L0
  constraint perpendicular L0 L1
  constraint parallel L0 L2
  constraint parallel L1 L3
  constraint coincident L4 origin
  constraint coincident L5 origin
  measures "d1" distance of L1.end L2.end
  measures "d2" distance of L0.end L1.end
extrude "Extrusion1" add sketch "Skizze1" along normal blind 5
sketch "Skizze2" plane through (0, 0, 5) normal (0, 0, 1) x (-1, 0, 0)
  line L0 (20, 40) -> (-20, 40)
  line L1 (-20, 40) -> (-20, -40)
  line L2 (-20, -40) -> (20, -40)
  line L3 (20, -40) -> (20, 40)
  line L4 (0, 0) -> (0, 20)
  dimension "d5" = 20
  constraint coincident L4.start origin
  constraint vertical L4
  measures "d5" distance of L0 L4.end
hole "Bohrung1" at (0, -20, 5) direction (0, 0, -1) diameter 7 depth 100 tip angle 118
fillet "Abrundung1" radius 2 4 edges at (-20, -40, 2.5) (20, -40, 2.5) (-20, 40, 2.5) (20, 40, 2.5)
sketch "Skizze3" plane through (0, 0, 5) normal (0, 0, 1) x (-1, 0, 0)
  circle A0 centre (0, 20) radius 3.5
  arc A1 (-20, -38) -> (-18, -40) centre (-18, -38) ccw
  line L0 (-18, -40) -> (18, -40)
  arc A2 (18, -40) -> (20, -38) centre (18, -38) ccw
  line L1 (20, -38) -> (20, 38)
  arc A3 (20, 38) -> (18, 40) centre (18, 38) ccw
  line L2 (18, 40) -> (-18, 40)
  arc A4 (-18, 40) -> (-20, 38) centre (-18, 38) ccw
  line L3 (-20, 38) -> (-20, -38)

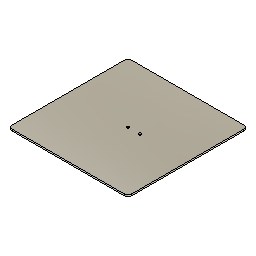
design "ScalePlate"
Autodesk Fusion 360 part; units mm, degrees
sketch "Skizze1" plane through (0, 0, 0) normal (0, 0, 1) x (1, 0, 0)
  line L0 (-75, 75) -> (75, 75)
  line L1 (75, 75) -> (75, -75)
  line L2 (75, -75) -> (-75, -75)
  line L3 (-75, -75) -> (-75, 75)
  line L4 (-75, 75) -> (75, -75) construction
  line L5 (75, 75) -> (-75, -75) construction
  dimension "d1" = 150
  dimension "d2" = 150
  constraint horizontal L0
  constraint perpendicular L0 L1
  constraint parallel L0 L2
  constraint parallel L1 L3
  constraint coincident L4 origin
  constraint coincident L5 origin
  measures "d1" distance of L1.end L2.end
  measures "d2" distance of L0.end L1.end
extrude "Extrusion1" add sketch "Skizze1" along normal blind 2
sketch "Skizze3" plane through (0, 0, 2) normal (0, 0, 1) x (-1, 0, 0)
  line L0 (75, -75) -> (75, 75)
  line L1 (-75, 75) -> (-75, -75)
  line L2 (-75, -75) -> (75, -75)
  line L3 (0, 0) -> (-15, 0)
  dimension "d17" = 15
  constraint horizontal L3
  constraint coincident origin L3
  constraint coincident L3.start origin
  measures "d17" distance of L3.start L3.end
hole "Bohrung1" at (15, 0, 2) at (0, 0, 2) direction (0, 0, -1) diameter 3.332 depth 10 tip angle 118
thread "Gewinde1" "ISO Metric profile 4.0 M4x0.7 6H"
fillet "Abrundung1" radius 5 4 edges at (75, -75, 1) (-75, -75, 1) (75, 75, 1) (-75, 75, 1)
sketch "Skizze4" plane through (0, 0, 2) normal (0, 0, 1) x (-1, 0, 0)
  arc A0 (70, -75) -> (75, -70) centre (70, -70) ccw
  line L0 (75, -70) -> (75, 70)
  arc A1 (75, 70) -> (70, 75) centre (70, 70) ccw
  line L1 (70, 75) -> (-70, 75)
  arc A2 (-70, 75) -> (-75, 70) centre (-70, 70) ccw
  line L2 (-75, 70) -> (-75, -70)
  arc A3 (-75, -70) -> (-70, -75) centre (-70, -70) ccw
  line L3 (-70, -75) -> (70, -75)
  circle A4 centre (-15, 0) radius 1.666
  circle A5 centre (0, 0) radius 1.666
named bodies: "ScalePlate"

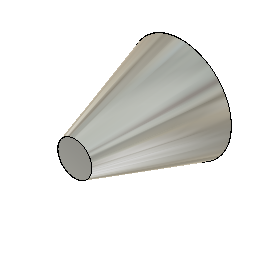
design "Trichter_groß"
Autodesk Fusion 360 part; units mm, degrees
sketch "Skizze1" plane through (0, 0, 0) normal (1, 0, 0) x (0, 1, 0)
  line L0 (-580, 70) -> (-580, 0)
  line L1 (-580, 0) -> (0, 0)
  line L2 (0, 250) -> (0, 0)
  line L3 (-580, 70) -> (0, 250)
  line L4 (-230, 0) -> (-230, 178.6207)
  line L5 (-530, 0) -> (-530, 85.5172)
  dimension "d3" = 250
  dimension "d4" = 70
  dimension "d5" = 580
  dimension "d8" = 230
  dimension "d9" = 530
  constraint vertical L0
  constraint perpendicular L0 L1
  constraint perpendicular L1 L2
  constraint coincident L1.end L2
  constraint coincident L2.end L1
  constraint coincident L1 L4.start
  constraint coincident L3 L4.end
  constraint perpendicular L1 L4
  constraint coincident L1 L5.start
  constraint coincident L3 L5.end
  constraint perpendicular L1 L5
  measures "d3" distance of L1.end L2.start
  measures "d4" vertical distance of L1.end L0.start
  measures "d5" distance of L1.end L0
  measures "d8" distance of L2 L4
  measures "d9" distance of L2 L5
revolve "Drehen1" add sketch "Skizze1" angle 360 about axis through (0, -580, 0) along (0, 1, 0) contours L1 L3 L4 L5 | L1 L2 L3 L4
shell "Schale1" thickness 1 removed faces 1 at (54.8247, 0, 36.3167)

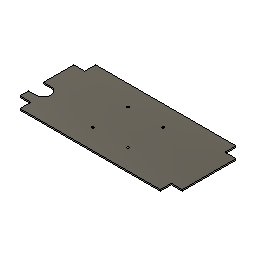
design "ScaleFramePlate"
Autodesk Fusion 360 part; units mm, degrees
sketch "Skizze1" plane through (0, 0, 0) normal (0, 0, 1) x (1, 0, 0)
  line L0 (-300, 140) -> (300, 140)
  line L1 (300, 140) -> (300, -140)
  line L2 (300, -140) -> (-300, -140)
  line L3 (-300, -140) -> (-300, 140)
  line L4 (-300, 140) -> (300, -140) construction
  line L5 (300, 140) -> (-300, -140) construction
  dimension "d1" = 600
  dimension "d2" = 280
  constraint horizontal L0
  constraint perpendicular L0 L1
  constraint parallel L0 L2
  constraint parallel L1 L3
  constraint coincident L4 origin
  constraint coincident L5 origin
  measures "d1" distance of L1.end L2.end
  measures "d2" distance of L0.end L1.end
extrude "Extrusion1" add sketch "Skizze1" along normal blind 5
sketch "Skizze2" plane through (0, 0, 5) normal (0, 0, 1) x (-1, 0, 0)
  line L0 (300, 140) -> (-300, 140)
  line L1 (-300, 140) -> (-300, -140)
  line L2 (-300, -140) -> (300, -140)
  line L3 (300, -140) -> (300, 140)
  line L4 (259.5, -99.5) -> (-259.5, -99.5)
  line L5 (-259.5, -99.5) -> (-259.5, 99.5)
  line L6 (-259.5, 99.5) -> (259.5, 99.5)
  line L7 (259.5, 99.5) -> (259.5, -99.5)
  line L8 (259.5, -99.5) -> (-259.5, 99.5) construction
  line L9 (-259.5, -99.5) -> (259.5, 99.5) construction
  line L10 (300, -140) -> (259.5, -140)
  line L11 (259.5, -140) -> (259.5, -99.5)
  line L12 (259.5, -99.5) -> (300, -99.5)
  line L13 (300, -99.5) -> (300, -140)
  line L14 (300, 140) -> (259.5, 140)
  line L15 (259.5, 140) -> (259.5, 99.5)
  line L16 (259.5, 99.5) -> (300, 99.5)
  line L17 (300, 99.5) -> (300, 140)
  line L18 (-300, 140) -> (-259.5, 140)
  line L19 (-259.5, 140) -> (-259.5, 99.5)
  line L20 (-259.5, 99.5) -> (-300, 99.5)
  line L21 (-300, 99.5) -> (-300, 140)
  line L22 (-300, -140) -> (-259.5, -140)
  line L23 (-259.5, -140) -> (-259.5, -99.5)
  line L24 (-259.5, -99.5) -> (-300, -99.5)
  line L25 (-300, -99.5) -> (-300, -140)
  dimension "d5" = 40.5
  dimension "d6" = 40.5
  constraint horizontal L4
  constraint perpendicular L4 L5
  constraint parallel L4 L6
  constraint parallel L5 L7
  constraint coincident L8 origin
  constraint coincident L9 origin
  constraint horizontal L10
  constraint vertical L11
  constraint horizontal L12
  constraint vertical L13
  constraint coincident L2.end L3.start
  constraint horizontal L14
  constraint vertical L15
  constraint horizontal L16
  constraint vertical L17
  constraint coincident L0.start L3.end
  constraint horizontal L18
  constraint vertical L19
  constraint horizontal L20
  constraint vertical L21
  constraint coincident L0.end L1.start
  constraint horizontal L22
  constraint vertical L23
  constraint horizontal L24
  constraint vertical L25
  constraint coincident L1.end L2.start
  measures "d5" distance of L3 L7
  measures "d6" distance of L2 L4
extrude "Extrusion2" cut sketch "Skizze2" against normal up to surface (5 mm away) contours L0 L3 L14 L15 L16 L17 | L0 L1 L18 L19 L20 L21 | L2 L3 L10 L11 L12 L13 | L1 L2 L22 L23 L24 L25
sketch "Skizze3" plane through (0, 0, 5) normal (0, 0, 1) x (-1, 0, 0)
  line L0 (259.5, 99.5) -> (259.5, 140)
  line L1 (259.5, 140) -> (-259.5, 140)
  line L2 (-259.5, 140) -> (-259.5, 99.5)
  line L3 (-259.5, 99.5) -> (-300, 99.5)
  line L4 (-300, 99.5) -> (-300, -99.5)
  line L5 (-300, -99.5) -> (-259.5, -99.5)
  line L6 (-259.5, -99.5) -> (-259.5, -140)
  line L7 (-259.5, -140) -> (259.5, -140)
  line L8 (259.5, -140) -> (259.5, -99.5)
  line L9 (259.5, -99.5) -> (300, -99.5)
  line L10 (300, -99.5) -> (300, 99.5)
  line L11 (300, 99.5) -> (259.5, 99.5)
  line L12 (65, -65) -> (-65, -65)
  line L13 (-65, -65) -> (-65, 65)
  line L14 (-65, 65) -> (65, 65)
  line L15 (65, 65) -> (65, -65)
  line L16 (65, -65) -> (-65, 65) construction
  line L17 (-65, -65) -> (65, 65) construction
  dimension "d9" = 130
  dimension "d10" = 130
  constraint horizontal L12
  constraint perpendicular L12 L13
  constraint parallel L12 L14
  constraint parallel L13 L15
  constraint coincident L16 origin
  constraint coincident L17 origin
  measures "d9" distance of L13.end L14.end
  measures "d10" distance of L12.end L13.end
hole "Bohrung1" at (-65, 65, 5) at (65, 65, 5) at (-65, -65, 5) at (65, -65, 5) direction (0, 0, -1) diameter 8.5 depth 100 tip angle 118
fillet "Abrundung1" radius 1 12 edges at (-300, -99.5, 2.5) (-259.5, -99.5, 2.5) (-259.5, -140, 2.5) (259.5, -99.5, 2.5) (300, -99.5, 2.5) (259.5, -140, 2.5) (259.5, 140, 2.5) (259.5, 99.5, 2.5) (300, 99.5, 2.5) (-259.5, 140, 2.5) (-259.5, 99.5, 2.5) (-300, 99.5, 2.5)
sketch "Skizze6" plane through (0, 0, 5) normal (0, 0, 1) x (-1, 0, 0)
  arc A0 (299, -99.5) -> (300, -98.5) centre (299, -98.5) ccw
  line L0 (300, -98.5) -> (300, 98.5)
  arc A1 (300, 98.5) -> (299, 99.5) centre (299, 98.5) ccw
  line L1 (299, 99.5) -> (260.5, 99.5)
  arc A2 (259.5, 100.5) -> (260.5, 99.5) centre (260.5, 100.5) ccw
  line L2 (259.5, 100.5) -> (259.5, 139)
  arc A3 (259.5, 139) -> (258.5, 140) centre (258.5, 139) ccw
  line L3 (258.5, 140) -> (-258.5, 140)
  arc A4 (-258.5, 140) -> (-259.5, 139) centre (-258.5, 139) ccw
  line L4 (-259.5, 139) -> (-259.5, 100.5)
  arc A5 (-260.5, 99.5) -> (-259.5, 100.5) centre (-260.5, 100.5) ccw
  line L5 (-260.5, 99.5) -> (-299, 99.5)
  arc A6 (-299, 99.5) -> (-300, 98.5) centre (-299, 98.5) ccw
  line L6 (-300, 98.5) -> (-300, -98.5)
  arc A7 (-300, -98.5) -> (-299, -99.5) centre (-299, -98.5) ccw
  line L7 (-299, -99.5) -> (-260.5, -99.5)
  arc A8 (-259.5, -100.5) -> (-260.5, -99.5) centre (-260.5, -100.5) ccw
  line L8 (-259.5, -100.5) -> (-259.5, -139)
  arc A9 (-259.5, -139) -> (-258.5, -140) centre (-258.5, -139) ccw
  line L9 (-258.5, -140) -> (258.5, -140)
  arc A10 (258.5, -140) -> (259.5, -139) centre (258.5, -139) ccw
  line L10 (259.5, -139) -> (259.5, -100.5)
  arc A11 (260.5, -99.5) -> (259.5, -100.5) centre (260.5, -100.5) ccw
  line L11 (260.5, -99.5) -> (299, -99.5)
  circle A12 centre (65, 65) radius 4.25
  circle A13 centre (65, -65) radius 4.25
  circle A14 centre (-65, -65) radius 4.25
  circle A15 centre (-65, 65) radius 4.25
  line L12 (331.3546, 12.5) -> (272.5, 12.5)
  line L13 (272.5, 12.5) -> (272.5, 67.5)
  line L14 (272.5, 67.5) -> (331.3546, 67.5)
  line L15 (331.3546, 67.5) -> (331.3546, 12.5)
  circle A16 centre (272.5, 40) radius 27.5
  dimension "d19" = 55
  dimension "d20" = 100
  dimension "d21" = 27.5
  constraint horizontal L12
  constraint vertical L13
  constraint horizontal L14
  constraint vertical L15
  constraint tangent L12 A16
  constraint tangent L14 A16
  constraint coincident L13 A16.centre
  measures "d19" diameter of A16
  measures "d20" distance of L3 A16.centre
  measures "d21" distance of L0 A16.centre
extrude "Extrusion3" cut sketch "Skizze6" against normal blind 10 contours L0 L12 A16 | L0 L14 A16 | L13 A16 | L13 A16